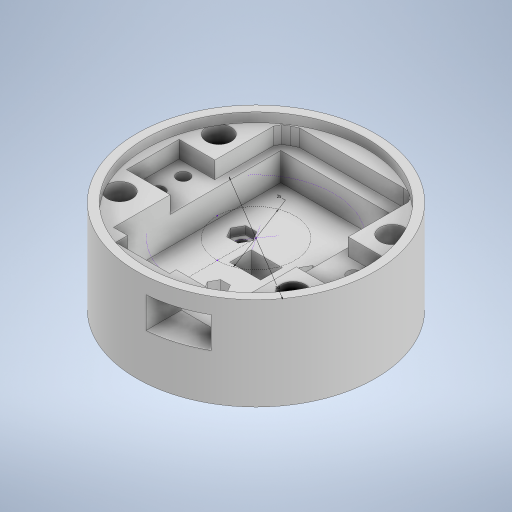
# Autodesk Inventor part: UR5_Mechanical_drawing
Saved by Autodesk Inventor 2024 (Build 280153000, 153)
## iProperties
Created: 2023-12-11
Part Number: UR5_Mechanical_drawing
Material: Generic
Document SubType Name: Modeling
Designer: Zakaria
Density: 1 g/cm^3
Appearance: Default
Author: Zakaria
## iProperties of the stored document Tiago_UR5_Mechanical_drawing_3DPrint.ipt
Created: 2023-12-13
Part Number: Tiago_UR5_Mechanical_drawing_3DPrint
Material: Generic
Document SubType Name: Modeling
Designer: Jeroen
Density: 1 g/cm^3
Appearance: Default
Author: Jeroen
Autodesk Inventor part; units mm, degrees
ref_plane "YZ Plane" through (0, 0, 0) normal (1, 0, 0) x (0, 1, 0)
ref_plane "XZ Plane" through (0, 0, 0) normal (0, 1, 0) x (-1, 0, 0)
ref_plane "XY Plane" through (0, 0, 0) normal (0, 0, 1) x (1, 0, 0)
sketch "Sketch1" plane through (0, 0, 0) normal (0, 1, 0) x (-1, 0, 0)
  circle A0 centre (0, 0) radius 38.5
  dimension "d0" = 77
  constraints: 1 centre point, 1 coincident
  measures "d0" diameter of A0
extrude "Extrusion1" add sketch "Sketch1" along normal blind 20
sketch "Sketch2" plane through (0, 20, 0) normal (0, 1, 0) x (1, 0, 0)
  circle A0 centre (0, 0) radius 25 construction
  point P0 (0, 0)
  dimension "d3" = 50
  constraints: 1 centre point, 1 coincident
  measures "d3" diameter of A0
sketch "Sketch15" plane through (0, 20, 0) normal (0, 1, 0) x (1, 0, 0)
  circle A0 centre (0, 0) radius 12.5 construction
  line L0 (0, 0) -> (0, -23.0126) construction
  line L1 (-2.9, 4.25) -> (2.9, -4.25) construction
  line L2 (2.9, 4.25) -> (-2.9, -4.25) construction
  point P0 (0, -12.5)
  point P1 (0, -12.5)
  point P2 (-12.5, 0)
  point P3 (0, -12.5)
  dimension "d64" = 25
  constraints: 6 end point, 3 point on circle, 2 coincident, 2 midpoint, 1 centre point, 1 point on line, 1 vertical
  measures "d64" diameter of A0
hole "Hole2" at (0, 20, 12.5) direction (0, -1, 0) diameter 3.5 end through all
pattern_circular "Circular Pattern4" count 3 over 360 about axis through (0, 0, 0) along (0, 1, 0) of "Hole2"
sketch "Sketch27" plane through (0, 20, 0) normal (0, 1, 0) x (1, 0, 0)
  circle A0 centre (0, 0) radius 38.5
  dimension "d81" = 77
  constraints: 1 centre point, 1 coincident
  measures "d81" diameter of A0
extrude "Extrusion13" add sketch "Sketch27" along normal blind 10
sketch "Sketch28" plane through (0, 30, 0) normal (0, 1, 0) x (1, 0, 0)
  circle A0 centre (0, 0) radius 35.75
  dimension "d84" = 71.5
  constraints: 1 centre point, 1 coincident
  measures "d84" diameter of A0
extrude "Extrusion14" cut sketch "Sketch28" against normal blind 3
sketch "Sketch29" plane through (0, 27, 0) normal (0, 1, 0) x (1, 0, 0)
  circle A0 centre (-28, -16) radius 4
  line L0 (0, 0) -> (-47.1428, 0)
  line L1 (0, 0) -> (-34.1673, 0)
  circle A1 centre (-28, 16) radius 4
  line L2 (0, 0) -> (0, -26.8569)
  line L3 (0, 0) -> (0, 23.9063)
  circle A2 centre (28, 16) radius 4
  circle A3 centre (28, -16) radius 4
  dimension "d87" = 28
  dimension "d88" = 16
  dimension "d89" = 8
  constraints: 8 end point, 4 centre point, 3 symmetric about line, 2 vertical, 1 horizontal, 1 point on line, 3 other
  measures "d87" horizontal distance of L0.start A0.centre
  measures "d88" distance from line of L0 A0.centre
  measures "d89" diameter of A0
extrude "Extrusion15" cut sketch "Sketch29" against normal blind 15
sketch "Sketch31" plane through (0, 27, 0) normal (0, 1, 0) x (1, 0, 0)
  line L0 (-19, -27) -> (19, -27)
  line L1 (19, -27) -> (19, 27)
  line L2 (19, 27) -> (-19, 27)
  line L3 (-19, 27) -> (-19, -27)
  line L4 (-19, -27) -> (19, 27) construction
  line L5 (19, -27) -> (-19, 27) construction
  point P0 (0, 0)
  dimension "d95" = 38
  dimension "d96" = 54
  constraints: 12 end point, 2 midpoint, 2 parallel, 1 horizontal, 1 perpendicular
  measures "d95" distance of L2.end L1.end
  measures "d96" distance of L1.end L0.end
extrude "Extrusion17" cut sketch "Sketch31" against normal blind 14.5
sketch "Sketch32" plane through (0, 0, 0) normal (0, -1, 0) x (1, 0, 0)
  point P0 (0, 0)
sketch "Sketch34" plane through (0, 27, 0) normal (0, 1, 0) x (1, 0, 0)
  circle A0 centre (-27.5, 4) radius 2
  line L0 (0, 0) -> (-42.522, 0)
  line L1 (-19, -27) -> (-19, 27) projected
  line L2 (0, 0) -> (-33.389, 0)
  circle A1 centre (-27.5, -4) radius 2
  line L3 (0, 0) -> (0, 41.3925)
  circle A2 centre (27.5, 4) radius 2
  line L4 (0, 0) -> (53.9479, 0)
  circle A3 centre (27.5, -4) radius 2
  dimension "d105" = 4
  dimension "d108" = 55
  dimension "d143" = 4
  constraints: 8 end point, 4 centre point, 3 symmetric about line, 2 horizontal, 1 point on line, 1 vertical, 3 other
  measures "d105" distance from line of L0 A0.centre
  measures "d108" distance of A2.centre A0.centre
  measures "d143" diameter of A3
extrude "Extrusion19" cut sketch "Sketch34" against normal blind 11.2
sketch "Sketch36" plane through (0, 27, 0) normal (0, 1, 0) x (1, 0, 0)
  line L0 (-20.9695, 21.8887) -> (-20.9696, 22.2063) construction
  line L1 (-20.9696, 22.2063) -> (-21.4696, 22.2061) construction
  line L2 (-21.4696, 22.2061) -> (-21.4696, 22.2061) construction
  line L3 (-21.4696, 22.2061) -> (-21.4696, 10.3125)
  line L4 (-24.9291, 8.1862) -> (-30.4516, 8.1862)
  line L5 (-30.4516, 8.1862) -> (-33.0317, 8.1862)
  line L6 (-33.0317, 8.1862) -> (-33.0317, -8.7514)
  line L7 (-33.0317, -8.7514) -> (-19, -8.7514)
  line L8 (-19, -8.7514) -> (-19, -24.3814)
  line L9 (2.9605, -30.8496) -> (2.9605, -28.7229)
  line L10 (2.9605, -28.7229) -> (18.1667, -28.7229)
  line L11 (18.1667, -28.7229) -> (20.4983, -28.7229)
  line L12 (20.4983, -28.7229) -> (21.5481, -28.0989)
  line L13 (21.5481, -28.0989) -> (21.5481, -24.3615)
  line L14 (21.5481, -24.3615) -> (21.5481, -11.5765)
  line L15 (26.016, -8.5347) -> (32.6917, -8.5347)
  line L16 (32.6917, -8.5347) -> (32.6917, 8.2274)
  line L17 (32.6917, 8.2274) -> (26.003, 8.2274)
  line L18 (21.535, 10.6207) -> (21.535, 27.634)
  line L19 (21.535, 27.634) -> (21.035, 28.4759)
  line L20 (21.035, 28.4759) -> (18.8556, 30.5832)
  line L21 (18.8556, 30.5832) -> (16.7875, 30.8605)
  line L22 (16.7875, 30.8605) -> (14.643, 30.8605)
  line L23 (14.643, 30.8605) -> (7.59, 30.8605)
  line L24 (7.59, 30.8605) -> (-10.2321, 30.8605)
  line L25 (-10.2321, 30.8605) -> (-16.8238, 30.8605)
  line L26 (-16.8238, 30.8605) -> (-18.7434, 29.9175)
  line L27 (-18.7434, 29.9175) -> (-20.5678, 28.834)
  line L28 (-20.5678, 28.834) -> (-21.4696, 27.1504)
  line L29 (-21.4696, 27.1504) -> (-21.4696, 22.2061)
  line L30 (-14.4477, -30.8496) -> (-14.4477, -27)
  line L31 (-14.4477, -27) -> (-19, -27)
  line L32 (-19, -27) -> (-19, -24.3814)
  line L33 (2.9605, -30.8496) -> (-14.4477, -30.8496)
  line L34 (-21.4696, 10.3125) -> (-21.4696, 8.1862)
  line L35 (-21.4696, 8.1862) -> (-24.9291, 8.1862)
  line L36 (21.535, 10.6207) -> (21.535, 8.2274)
  line L37 (21.535, 8.2274) -> (26.003, 8.2274)
  line L38 (26.016, -8.5347) -> (21.5481, -8.5347)
  line L39 (21.5481, -8.5347) -> (21.5481, -11.5765)
  point P0 (0, 0)
  point P1 (-30.965, -5.065)
  dimension "d117" = 0.5
  constraints: 80 end point, 13 perpendicular, 5 parallel, 5 point on line, 4 vertical, 3 horizontal, 1 other
  measures "d117" distance of L0.end L1.end
extrude "Extrusion20" cut sketch "Sketch36" against normal blind 5.5
sketch "Sketch41" plane through (0, 12.5, 0) normal (0, 1, 0) x (1, 0, 0)
  circle A0 centre (0, -12.5) radius 1.75
  line L0 (1.494, -9.7636) -> (3.1168, -12.4257)
  line L1 (3.1168, -12.4257) -> (1.6228, -15.1621)
  line L2 (1.6228, -15.1621) -> (-1.494, -15.2364)
  line L3 (-1.494, -15.2364) -> (-3.1168, -12.5743)
  line L4 (-3.1168, -12.5743) -> (-1.6228, -9.8379)
  line L5 (-1.6228, -9.8379) -> (1.494, -9.7636)
  point P0 (0, 0)
  dimension "d119" = 5.4
  constraints: 12 end point, 1 centre point, 1 coincident, 13 other
  measures "d119" distance between parallel lines of L5 L2
extrude "Extrusion21" cut sketch "Sketch41" against normal blind 3.5
sketch "Sketch42" plane through (0, 12.5, 0) normal (0, 1, 0) x (1, 0, 0)
  circle A0 centre (-10.8253, 6.25) radius 1.75 projected
  line L0 (-8.531, 7.9175) -> (-8.2341, 5.0968)
  line L1 (-8.2341, 5.0968) -> (-10.5284, 3.4294)
  line L2 (-10.5284, 3.4294) -> (-13.1196, 4.5825)
  line L3 (-13.1196, 4.5825) -> (-13.4165, 7.4032)
  line L4 (-13.4165, 7.4032) -> (-11.1222, 9.0706)
  line L5 (-11.1222, 9.0706) -> (-8.531, 7.9175)
  point P0 (0, 0)
  constraints: 12 end point, 1 coincident, 13 other
sketch "Sketch43" plane through (0, 12.5, 0) normal (0, 1, 0) x (1, 0, 0)
  circle A0 centre (-10.8253, 6.25) radius 1.75 projected
  line L0 (-8.9933, 3.1878) -> (-12.5612, 3.1323)
  line L1 (-12.5612, 3.1323) -> (-14.3933, 6.1945)
  line L2 (-14.3933, 6.1945) -> (-12.6574, 9.3122)
  line L3 (-12.6574, 9.3122) -> (-9.0894, 9.3677)
  line L4 (-9.0894, 9.3677) -> (-7.2574, 6.3055)
  line L5 (-7.2574, 6.3055) -> (-8.9933, 3.1878)
  point P0 (0, 0)
  point P1 (-8.1253, 4.7467)
  point P2 (-13.5253, 7.7533)
  dimension "d122" = 5.4
  constraints: 12 end point, 2 midpoint, 1 coincident, 13 other
  measures "d122" horizontal distance of point (-8.125, 4.747) point (-13.525, 7.753)
extrude "Extrusion22" cut sketch "Sketch43" against normal blind 2.6
sketch "Sketch44" plane through (0, 12.5, 0) normal (0, 1, 0) x (1, 0, 0)
  circle A0 centre (10.8253, 6.25) radius 1.75 projected
  line L0 (13.943, 6.2392) -> (12.3748, 3.5446)
  line L1 (12.3748, 3.5446) -> (9.2572, 3.5554)
  line L2 (9.2572, 3.5554) -> (7.7076, 6.2608)
  line L3 (7.7076, 6.2608) -> (9.2758, 8.9554)
  line L4 (9.2758, 8.9554) -> (12.3935, 8.9446)
  line L5 (12.3935, 8.9446) -> (13.943, 6.2392)
  point P0 (0, 0)
  dimension "d125" = 5.4
  constraints: 12 end point, 1 coincident, 13 other
  measures "d125" distance between parallel lines of L5 L2
extrude "Extrusion23" cut sketch "Sketch44" against normal blind 3.5
sketch "Sketch45" plane through (0, 12.5, 0) normal (0, 1, 0) x (1, 0, 0)
  line L0 (-5, -3.5) -> (5, -3.5)
  line L1 (5, -3.5) -> (5, 3.5)
  line L2 (5, 3.5) -> (-5, 3.5)
  line L3 (-5, 3.5) -> (-5, -3.5)
  line L4 (-5, -3.5) -> (5, 3.5) construction
  line L5 (5, -3.5) -> (-5, 3.5) construction
  point P0 (0, 0)
  dimension "d132" = 10
  dimension "d133" = 7
  constraints: 12 end point, 2 midpoint, 2 parallel, 1 horizontal, 1 perpendicular
  measures "d132" distance of L2.end L1.end
  measures "d133" distance of L1.end L0.end
extrude "Extrusion25" cut sketch "Sketch45" against normal through all
sketch "Sketch46" plane through (19, 12.5, 27) normal (0, 0, -1) x (-1, 0, 0)
  point P0 (19, -12.5)
sketch "Sketch47" plane through (19, 12.5, 27) normal (0, 0, -1) x (-1, 0, 0)
  line L0 (0.0055, 2.3292) -> (16.1055, 2.3292)
  line L1 (16.1055, 2.3292) -> (16.1055, 12.3292)
  line L2 (16.1055, 12.3292) -> (0.0055, 12.3292)
  line L3 (0.0055, 12.3292) -> (0.0055, 2.3292)
  point P0 (19, -12.5)
  point P1 (8.0555, 2.3292)
  dimension "d139" = 16.1
  dimension "d140" = 10
  constraints: 8 end point, 2 parallel, 1 horizontal, 1 midpoint, 1 perpendicular
  measures "d139" distance between parallel lines of L3 L1
  measures "d140" distance from line of L2 point (8.055, 2.329)
extrude "Extrusion26" cut sketch "Sketch47" against normal through all
body "Solid1"
